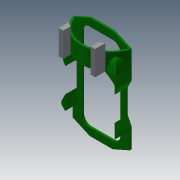
# Autodesk Inventor part: podvozek_dibond
Saved by Autodesk Inventor 2013 (Build 170138000, 138)
## iProperties
Created: 2012-09-03
Part Number: podvozek_dibond
Material: Generic
Document SubType Name: Modeling
Designer: idle-rug
Density: 1 g/cm^3
Author: idle-rug
Autodesk Inventor part; units mm, degrees
ref_plane "YZ Plane" through (0, 0, 0) normal (1, 0, 0) x (0, 1, 0)
ref_plane "XZ Plane" through (0, 0, 0) normal (0, 1, 0) x (-1, 0, 0)
ref_plane "XY Plane" through (0, 0, 0) normal (0, 0, 1) x (1, 0, 0)
sketch "Sketch1" plane through (0, 0, 0) normal (0, 1, 0) x (-1, 0, 0)
  circle A0 centre (24.1, 110.65) radius 0.25
  circle A1 centre (-70.5, 110.65) radius 0.25
  circle A2 centre (-45.6, 89.15) radius 0.25
  circle A3 centre (0, 67.65) radius 0.25
  circle A4 centre (70.5, 42.15) radius 0.25
  circle A5 centre (32.15, 17.15) radius 0.25
  circle A6 centre (60.5, -17.65) radius 0.25
  circle A7 centre (-60.5, -17.65) radius 0.25
  circle A8 centre (24.1, -67.65) radius 0.25
  circle A9 centre (-70.5, -67.65) radius 0.25
  circle A10 centre (-45.6, -89.15) radius 0.25
  circle A11 centre (0, -110.65) radius 0.25
  circle A12 centre (-70.5, -110.65) radius 0.25
  circle A13 centre (70.5, -110.65) radius 0.25
  circle A14 centre (45.6, -89.15) radius 0.25
  circle A15 centre (-24.1, -67.65) radius 0.25
  circle A16 centre (70.5, -67.65) radius 0.25
  circle A17 centre (0, -17.65) radius 0.25
  circle A18 centre (-32.15, 17.15) radius 0.25
  circle A19 centre (-70.5, 42.15) radius 0.25
  circle A20 centre (-70.5, 67.65) radius 0.25
  circle A21 centre (70.5, 67.65) radius 0.25
  circle A22 centre (45.6, 89.15) radius 0.25
  circle A23 centre (-24.1, 110.65) radius 0.25
  circle A24 centre (70.5, 110.65) radius 0.25
  line L0 (75.5, -115.65) -> (75.5, -62.65)
  line L1 (75.5, -62.65) -> (65.5, -42.65)
  line L2 (65.5, -42.65) -> (65.5, 22.15)
  line L3 (65.5, 22.15) -> (75.5, 42.15)
  line L4 (75.5, 42.15) -> (75.5, 115.65)
  line L5 (75.5, 115.65) -> (30.5, 135.65)
  line L6 (30.5, 135.65) -> (-30.5, 135.65)
  line L7 (-30.5, 135.65) -> (-75.5, 115.65)
  line L8 (-75.5, 115.65) -> (-75.5, 42.15)
  line L9 (-75.5, 42.15) -> (-65.5, 22.15)
  line L10 (-65.5, 22.15) -> (-65.5, -42.65)
  line L11 (-65.5, -42.65) -> (-75.5, -62.65)
  line L12 (-75.5, -62.65) -> (-75.5, -115.65)
  line L13 (-75.5, -115.65) -> (-30.5, -135.65)
  line L14 (-30.5, -135.65) -> (30.5, -135.65)
  line L15 (30.5, -135.65) -> (75.5, -115.65)
  circle A25 centre (0, -110.65) radius 2
  circle A26 centre (70.5, -110.65) radius 2
  circle A27 centre (-70.5, -110.65) radius 2
  circle A28 centre (45.6, -89.15) radius 2
  circle A29 centre (-45.6, -89.15) radius 2
  circle A30 centre (70.5, -67.65) radius 2
  circle A31 centre (24.1, -67.65) radius 2
  circle A32 centre (-24.1, -67.65) radius 2
  circle A33 centre (-70.5, -67.65) radius 2
  circle A34 centre (60.5, -17.65) radius 2
  circle A35 centre (0, -17.65) radius 2
  circle A36 centre (-32.15, 17.15) radius 2
  circle A37 centre (-60.5, -17.65) radius 2
  circle A38 centre (32.15, 17.15) radius 2
  circle A39 centre (70.5, 42.15) radius 2
  circle A40 centre (-70.5, 42.15) radius 2
  circle A41 centre (-70.5, 67.65) radius 2
  circle A42 centre (0, 67.65) radius 2
  circle A43 centre (70.5, 67.65) radius 2
  circle A44 centre (45.6, 89.15) radius 2
  circle A45 centre (-45.6, 89.15) radius 2
  circle A46 centre (-70.5, 110.65) radius 2
  circle A47 centre (-24.1, 110.65) radius 2
  circle A48 centre (24.1, 110.65) radius 2
  circle A49 centre (70.5, 110.65) radius 2
  point P0 (0, 0)
  point P1 (0, 0)
  dimension "d0" = 4
  dimension "d1" = 4
  dimension "d2" = 4
  dimension "d3" = 4
  dimension "d4" = 4
  dimension "d5" = 4
  dimension "d6" = 4
  dimension "d7" = 4
  dimension "d8" = 4
  dimension "d9" = 4
  dimension "d10" = 4
  dimension "d11" = 4
  dimension "d12" = 4
  dimension "d13" = 4
  dimension "d14" = 4
  dimension "d15" = 4
  dimension "d16" = 4
  dimension "d17" = 4
  dimension "d18" = 4
  dimension "d19" = 4
  dimension "d20" = 4
  dimension "d21" = 4
  dimension "d22" = 4
  dimension "d23" = 4
  dimension "d24" = 4
  constraints: 50 centre point, 32 end point, 25 coincident
  measures "d0" diameter of A25
  measures "d1" diameter of A26
  measures "d2" diameter of A27
  measures "d3" diameter of A28
  measures "d4" diameter of A29
  measures "d5" diameter of A30
  measures "d6" diameter of A31
  measures "d7" diameter of A32
  measures "d8" diameter of A33
  measures "d9" diameter of A34
  measures "d10" diameter of A35
  measures "d11" diameter of A36
  measures "d12" diameter of A37
  measures "d13" diameter of A38
  measures "d14" diameter of A39
  measures "d15" diameter of A40
  measures "d16" diameter of A41
  measures "d17" diameter of A42
  measures "d18" diameter of A43
  measures "d19" diameter of A44
  measures "d20" diameter of A45
  measures "d21" diameter of A46
  measures "d22" diameter of A47
  measures "d23" diameter of A48
  measures "d24" diameter of A49
extrude "Extrusion1" add sketch "Sketch1" along normal blind 2 contours L15 L14 L13 L12 L11 L10 L9 L8 L7 L6 L5 L4 L3 L2 L1 L0
sketch "Sketch2" plane through (0, 0, 0) normal (0, -1, 0) x (1, 0, 0)
  circle A0 centre (-70.5, 110.65) radius 2 projected
  circle A1 centre (-24.1, 110.65) radius 2 projected
  circle A2 centre (24.1, 110.65) radius 2 projected
  circle A3 centre (70.5, 110.65) radius 2 projected
  circle A4 centre (45.6, 89.15) radius 2 projected
  circle A5 centre (-45.6, 89.15) radius 2 projected
  circle A6 centre (-70.5, 67.65) radius 2 projected
  circle A7 centre (0, 67.65) radius 2 projected
  circle A8 centre (70.5, 67.65) radius 2 projected
  circle A9 centre (70.5, 42.15) radius 2 projected
  circle A10 centre (-70.5, 42.15) radius 2 projected
  circle A11 centre (-32.15, 17.15) radius 2 projected
  circle A12 centre (60.5, -17.65) radius 2 projected
  circle A13 centre (32.15, 17.15) radius 2 projected
  circle A14 centre (0, -17.65) radius 2 projected
  circle A15 centre (-60.5, -17.65) radius 2 projected
  circle A16 centre (70.5, -67.65) radius 2 projected
  circle A17 centre (24.1, -67.65) radius 2 projected
  circle A18 centre (-24.1, -67.65) radius 2 projected
  circle A19 centre (-70.5, -67.65) radius 2 projected
  circle A20 centre (45.6, -89.15) radius 2 projected
  circle A21 centre (-45.6, -89.15) radius 2 projected
  circle A22 centre (70.5, -110.65) radius 2 projected
  circle A23 centre (-70.5, -110.65) radius 2 projected
  circle A24 centre (0, -110.65) radius 2 projected
  line L0 (65.5, 22.15) -> (75.5, 42.15) projected
  line L1 (75.5, 42.15) -> (75.5, 115.65) projected
  line L2 (75.5, 115.65) -> (30.5, 135.65) projected
  line L3 (30.5, 135.65) -> (-30.5, 135.65) projected
  line L4 (-30.5, 135.65) -> (-75.5, 115.65) projected
  line L5 (-75.5, 115.65) -> (-75.5, 42.15) projected
  line L6 (-75.5, 42.15) -> (-65.5, 22.15) projected
  line L7 (-65.5, 22.15) -> (-65.5, -42.65) projected
  line L8 (-65.5, -42.65) -> (-75.5, -62.65) projected
  line L9 (-75.5, -62.65) -> (-75.5, -115.65) projected
  line L10 (-75.5, -115.65) -> (-30.5, -135.65) projected
  line L11 (-30.5, -135.65) -> (30.5, -135.65) projected
  line L12 (30.5, -135.65) -> (75.5, -115.65) projected
  line L13 (75.5, -115.65) -> (75.5, -62.65) projected
  line L14 (75.5, -62.65) -> (65.5, -42.65) projected
  line L15 (65.5, -42.65) -> (65.5, 22.15) projected
  point P0 (0, 0)
extrude "Extrusion2" add sketch "Sketch2" along normal blind 1.3
sketch "Sketch3" plane through (0, -1.3, 0) normal (0, -1, 0) x (1, 0, 0)
  circle A0 centre (0, -110.65) radius 2 projected
  circle A1 centre (-45.6, -89.15) radius 2 projected
  circle A2 centre (45.6, -89.15) radius 2 projected
  circle A3 centre (-24.1, -67.65) radius 2 projected
  circle A4 centre (24.1, -67.65) radius 2 projected
  circle A5 centre (0, 67.65) radius 2 projected
  circle A6 centre (-45.6, 89.15) radius 2 projected
  circle A7 centre (45.6, 89.15) radius 2 projected
  circle A8 centre (24.1, 110.65) radius 2 projected
  circle A9 centre (-24.1, 110.65) radius 2 projected
  line L0 (-75.5, 115.65) -> (-75.5, 42.15) projected
  line L1 (75.5, 115.65) -> (-75.5, 115.65)
  line L2 (-75.5, 115.65) -> (-75.5, 105.65)
  line L3 (-75.5, 105.65) -> (75.5, 105.65)
  line L4 (75.5, 105.65) -> (75.5, 115.65)
  line L5 (75.5, 72.65) -> (-75.5, 72.65)
  line L6 (-75.5, 72.65) -> (-75.5, 62.65)
  line L7 (-75.5, 62.65) -> (75.5, 62.65)
  line L8 (75.5, 62.65) -> (75.5, 72.65)
  line L9 (75.5, 72.65) -> (-75.5, 62.65) construction
  line L10 (-75.5, 72.65) -> (75.5, 62.65) construction
  line L11 (50.6, 115.65) -> (40.6, 115.65)
  line L12 (40.6, 115.65) -> (40.6, 62.65)
  line L13 (40.6, 62.65) -> (50.6, 62.65)
  line L14 (50.6, 62.65) -> (50.6, 115.65)
  line L15 (50.6, 115.65) -> (40.6, 62.65) construction
  line L16 (40.6, 115.65) -> (50.6, 62.65) construction
  line L17 (-40.6, 115.65) -> (-50.6, 115.65)
  line L18 (-50.6, 115.65) -> (-50.6, 62.65)
  line L19 (-50.6, 62.65) -> (-40.6, 62.65)
  line L20 (-40.6, 62.65) -> (-40.6, 115.65)
  line L21 (-40.6, 115.65) -> (-50.6, 62.65) construction
  line L22 (-50.6, 115.65) -> (-40.6, 62.65) construction
  line L23 (-75.5, -72.65) -> (75.5, -72.65)
  line L24 (75.5, -72.65) -> (75.5, -62.65)
  line L25 (75.5, -62.65) -> (-75.5, -62.65)
  line L26 (-75.5, -62.65) -> (-75.5, -72.65)
  line L27 (-75.5, -72.65) -> (75.5, -62.65) construction
  line L28 (75.5, -72.65) -> (-75.5, -62.65) construction
  line L29 (75.5, -105.65) -> (-75.5, -105.65)
  line L30 (-75.5, -105.65) -> (-75.5, -115.65)
  line L31 (-75.5, -115.65) -> (75.5, -115.65)
  line L32 (75.5, -115.65) -> (75.5, -105.65)
  line L33 (75.5, -105.65) -> (-75.5, -115.65) construction
  line L34 (-75.5, -105.65) -> (75.5, -115.65) construction
  line L35 (50.6, -62.65) -> (40.6, -62.65)
  line L36 (40.6, -62.65) -> (40.6, -115.65)
  line L37 (40.6, -115.65) -> (50.6, -115.65)
  line L38 (50.6, -115.65) -> (50.6, -62.65)
  line L39 (50.6, -62.65) -> (40.6, -115.65) construction
  line L40 (40.6, -62.65) -> (50.6, -115.65) construction
  line L41 (-40.6, -62.65) -> (-50.6, -62.65)
  line L42 (-50.6, -62.65) -> (-50.6, -115.65)
  line L43 (-50.6, -115.65) -> (-40.6, -115.65)
  line L44 (-40.6, -115.65) -> (-40.6, -62.65)
  line L45 (-40.6, -62.65) -> (-50.6, -115.65) construction
  line L46 (-50.6, -62.65) -> (-40.6, -115.65) construction
  line L47 (30.5, 135.65) -> (75.5, 115.65) projected
  line L48 (-50.6, 115.65) -> (50.6, 115.65)
  line L49 (50.6, 115.65) -> (50.6, -115.65)
  line L50 (50.6, -115.65) -> (-50.6, -115.65)
  line L51 (-50.6, -115.65) -> (-50.6, 115.65)
  point P0 (0, 0)
  point P1 (0, -67.65)
  dimension "d29" = 10
  dimension "d30" = 10
  dimension "d31" = 10
  dimension "d32" = 10
  dimension "d33" = 10
  dimension "d34" = 10
  constraints: 100 end point, 18 parallel, 14 midpoint, 9 horizontal, 9 perpendicular, 6 point on line
  measures "d29" distance of L2.end L1.end
  measures "d30" distance of L6.end L5.end
  measures "d31" distance of L13.end L12.end
  measures "d32" distance of L19.end L18.end
  measures "d33" distance of L37.end L36.end
  measures "d34" distance of L43.end L42.end
extrude "Extrusion3" cut sketch "Sketch3" against normal blind 3.3 contours A0 | A1 | A2 | A3 | A4 | A5 | A6 | A7 | A8 | A9 | L1 L20 L3 L18 | L3 L20 L5 L18 | L1 L12 L3 L20 | L5 L20 L7 L18 | L3 L12 L5 L20 | L1 L14 L3 L12 | L7 L49 L25 L51 | L5 L12 L7 L20 | L3 L14 L5 L12 | L25 L44 L23 L42 | L5 L14 L7 L12 | L25 L36 L23 L44 | L23 L44 L29 L42 | L25 L38 L23 L36 | L23 L36 L29 L44 | L29 L44 L31 L42 | L23 L38 L29 L36 | L29 L36 L31 L44 | L29 L38 L31 L36
fillet "Fillet1" radius 20 4 edges at (-50.6, 0.35, 115.65) (-50.6, 0.35, -115.65) (50.6, 0.35, -115.65) (50.6, 0.35, 115.65)
sketch "Sketch5" plane through (0, -1.3, 0) normal (0, -1, 0) x (1, 0, 0)
  circle A0 centre (-70.5, -110.65) radius 2 projected
  circle A1 centre (70.5, -110.65) radius 2 projected
  circle A2 centre (-70.5, -67.65) radius 2 projected
  circle A3 centre (70.5, -67.65) radius 2 projected
  circle A4 centre (-70.5, 42.15) radius 2 projected
  circle A5 centre (70.5, 42.15) radius 2 projected
  circle A6 centre (70.5, 67.65) radius 2 projected
  circle A7 centre (-70.5, 67.65) radius 2 projected
  circle A8 centre (70.5, 110.65) radius 2 projected
  circle A9 centre (-70.5, 110.65) radius 2 projected
  point P0 (0, 0)
extrude "Extrusion4" add sketch "Sketch5" against normal blind 3
sketch "Sketch6" plane through (0, 2, 0) normal (0, 1, 0) x (1, 0, 0)
  circle A0 centre (60.5, 17.65) radius 2 projected
  circle A1 centre (-60.5, 17.65) radius 2 projected
  point P0 (0, 0)
extrude "Extrusion5" add sketch "Sketch6" against normal blind 3.3
sketch "Sketch7" plane through (0, -1.3, 0) normal (0, -1, 0) x (1, 0, 0)
  line L0 (-30.6, 115.65) -> (30.6, 115.65) projected
  arc A0 (50.6, 95.65) -> (30.6, 115.65) centre (30.6, 95.65) ccw projected
  line L1 (50.6, 95.65) -> (50.6, -95.65) projected
  arc A1 (30.6, -115.65) -> (50.6, -95.65) centre (30.6, -95.65) ccw projected
  line L2 (30.6, -115.65) -> (-30.6, -115.65) projected
  arc A2 (-50.6, -95.65) -> (-30.6, -115.65) centre (-30.6, -95.65) ccw projected
  line L3 (-50.6, -95.65) -> (-50.6, 95.65) projected
  arc A3 (-30.6, 115.65) -> (-50.6, 95.65) centre (-30.6, 95.65) ccw projected
  line L4 (65.5, 22.15) -> (75.5, 42.15) projected
  line L5 (75.5, 42.15) -> (75.5, 115.65) projected
  line L6 (75.5, 115.65) -> (30.5, 135.65) projected
  line L7 (30.5, 135.65) -> (-30.5, 135.65) projected
  line L8 (-30.5, 135.65) -> (-75.5, 115.65) projected
  line L9 (-75.5, 115.65) -> (-75.5, 42.15) projected
  line L10 (-75.5, 42.15) -> (-65.5, 22.15) projected
  line L11 (-65.5, 22.15) -> (-65.5, -42.65) projected
  line L12 (-65.5, -42.65) -> (-75.5, -62.65) projected
  line L13 (-75.5, -62.65) -> (-75.5, -115.65) projected
  line L14 (-75.5, -115.65) -> (-30.5, -135.65) projected
  line L15 (-30.5, -135.65) -> (30.5, -135.65) projected
  line L16 (30.5, -135.65) -> (75.5, -115.65) projected
  line L17 (75.5, -115.65) -> (75.5, -62.65) projected
  line L18 (75.5, -62.65) -> (65.5, -42.65) projected
  line L19 (65.5, -42.65) -> (65.5, 22.15) projected
  point P0 (0, 0)
extrude "Extrusion6" add sketch "Sketch7" along normal blind 1.7
sketch "Sketch9" plane through (-30.5, 2, 135.65) normal (0, 0, 1) x (1, 0, 0)
  line L0 (106, 0) -> (101, 0)
  line L1 (-45, -5) -> (-40, -5)
  line L2 (106, -5) -> (101, -5)
  arc A0 (-45, -5) -> (106, -5) centre (30.5, 21.4528) ccw
  arc A1 (-40, -5) -> (101, -5) centre (30.5, 21.4528) ccw
  line L3 (106, -5) -> (101, -5)
  line L4 (-45, -5) -> (-40, -5)
  line L5 (-45, -5) -> (-35, -5) projected
  arc A2 (-40, -5) -> (101, -5) centre (30.5, 21.4528) ccw
  point P0 (-45, 0)
  dimension "d46" = 80
  constraints: 10 end point, 7 point on circle, 3 centre point, 3 concentric, 2 collinear, 1 midpoint
  measures "d46" radius of A0
extrude "Extrusion7" add sketch "Sketch9" against normal blind 65
sketch "Sketch10" plane through (-30.5, 2, 135.65) normal (0, 0, 1) x (1, 0, 0)
  arc A0 (-45, -5) -> (106, -5) centre (30.5, 21.4528) ccw projected
  line L0 (106, -5) -> (101, -5) projected
  arc A1 (-40, -5) -> (101, -5) centre (30.5, 21.4528) ccw projected
  line L1 (-40, -5) -> (-45, -5) projected
  point P0 (30.5, -2)
extrude "Extrusion8" cut sketch "Sketch10" against normal blind 20
sketch "Sketch11" plane through (0, -3, 0) normal (0, -1, 0) x (1, 0, 0)
  line L0 (75.5, -115.65) -> (75.5, -62.65) projected
  line L1 (75.5, -62.65) -> (65.5, -42.65) projected
  line L2 (-30.6, 115.65) -> (30.6, 115.65) projected
  line L3 (65.5, -42.65) -> (65.5, -95.65)
  line L4 (65.5, -95.65) -> (75.5, -95.65)
  line L5 (75.5, -62.65) -> (75.5, -95.65)
  line L6 (65.5, -42.65) -> (75.5, -62.65)
  line L7 (65.5, -42.65) -> (75.5, -62.65)
  line L8 (0, 0) -> (0, -83)
  line L9 (-65.5, -42.65) -> (-65.5, -95.65)
  line L10 (-65.5, -95.65) -> (-75.5, -95.65)
  line L11 (-75.5, -62.65) -> (-75.5, -95.65)
  line L12 (-65.5, -42.65) -> (-75.5, -62.65)
  dimension "d51" = 53
  constraints: 20 end point, 3 collinear, 2 perpendicular, 2 symmetric about line, 1 parallel, 1 point on line
  measures "d51" distance of L1.end L3.end
extrude "Extrusion9" add sketch "Sketch11" along normal blind 30
sketch "Sketch12" plane through (0, -3, 0) normal (0, -1, 0) x (1, 0, 0)
  line L0 (65.5, -95.65) -> (65.5, -42.65) projected
  line L1 (65.5, -42.65) -> (65.5, 22.15) projected
  line L2 (65.5, 22.15) -> (75.5, 42.15) projected
  line L3 (75.5, 42.15) -> (75.5, 70.65) projected
  line L4 (75.5, 70.65) -> (70.5, 70.65) projected
  line L5 (-75.5, 70.65) -> (-75.5, 42.15) projected
  line L6 (-75.5, 42.15) -> (-65.5, 22.15) projected
  line L7 (-65.5, 22.15) -> (-65.5, -42.65) projected
  line L8 (-65.5, -42.65) -> (-65.5, -95.65) projected
  line L9 (-65.5, -95.65) -> (-75.5, -95.65) projected
  line L10 (-75.5, -95.65) -> (-75.5, -115.65) projected
  line L11 (-75.5, -115.65) -> (-30.5, -135.65) projected
  line L12 (-30.5, -135.65) -> (30.5, -135.65) projected
  line L13 (30.5, -135.65) -> (75.5, -115.65) projected
  line L14 (75.5, -115.65) -> (75.5, -95.65) projected
  line L15 (75.5, -95.65) -> (65.5, -95.65) projected
  line L16 (-30.6, 115.65) -> (30.6, 115.65) projected
  line L17 (65.5, 23) -> (65.5, 70.65)
  line L18 (75.5, 70.65) -> (65.5, 70.65)
  line L19 (-75.5, 70.65) -> (75.5, 70.65) projected
  line L20 (75.5, 70.65) -> (75.5, 42.15)
  line L21 (75.5, 42.15) -> (65.5, 22.15)
  line L22 (65.5, 22) -> (65.5, 23)
  line L23 (-65.5, 22.15) -> (-75.5, 42.15)
  line L24 (-75.5, 42.15) -> (-75.5, 70.65)
  line L25 (-75.5, 70.65) -> (-65.5, 70.65)
  line L26 (-65.5, 70.65) -> (-65.5, 22.15)
  point P0 (-70.5, 70.65)
  point P1 (0, 0)
  constraints: 19 end point, 4 point on line, 3 collinear, 2 perpendicular, 1 parallel
extrude "Extrusion10" add sketch "Sketch12" along normal blind 30 contours L22 L17 L18 L4 L3 L2 | L26 L6 L5 L19
sketch "Sketch13" plane through (65.5, -33, 70.65) normal (0, 0, 1) x (1, 0, 0)
  arc A0 (0, 10.5208) -> (10, 30) centre (-65.5, 56.4528) ccw projected
  line L0 (0, 10.5208) -> (0, 0) projected
  line L1 (10, 0) -> (0, 0) projected
  line L2 (10, 30) -> (10, 0) projected
  point P0 (-65.5, 33)
extrude "Extrusion11" add sketch "Sketch13" along normal blind 35
sketch "Sketch14" plane through (0, -33, 0) normal (0, -1, 0) x (1, 0, 0)
  line L0 (-5, 75.5) -> (5, 75.5)
  line L1 (-75.5, 70.65) -> (-75.5, 62.65)
  line L2 (75.5, 62.65) -> (75.5, 70.65)
  line L3 (75.5, 42.15) -> (75.5, 105.65) projected
  arc A0 (-41.3014, 70.65) -> (-75.5, 45.15) centre (0, -20.4225) ccw
  arc A1 (75.5, 45.15) -> (41.3014, 70.65) centre (0, -20.4225) ccw
  line L4 (-75.5, 70.65) -> (-41.3014, 70.65)
  line L5 (41.3014, 70.65) -> (75.5, 70.65)
  line L6 (75.5, 70.65) -> (75.5, 45.15)
  line L7 (-75.5, 70.65) -> (-75.5, 45.15)
  point P0 (0, 0)
  point P1 (-75.5, 42.15)
  dimension "d58" = 3
  dimension "d59" = 3
  constraints: 14 end point, 5 point on circle, 2 centre point, 1 collinear, 1 perpendicular, 1 point on line
  measures "d58" distance of L3.start L6.end
  measures "d59" distance of point (-75.5, 42.15) L7.end
extrude "Extrusion12" add sketch "Sketch14" along normal blind 6.2
sketch "Sketch15" plane through (56.6841, -33, 70.65) normal (0, 0, 1) x (1, 0, 0)
  arc A0 (-6.9384, -6.2) -> (0, 0) centre (-56.6841, 56.4528) ccw projected
  line L0 (18.8159, -6.2) -> (-6.9384, -6.2) projected
  line L1 (18.8159, 0) -> (18.8159, -6.2) projected
  line L2 (8.8159, 0) -> (18.8159, 0) projected
  line L3 (8.8159, 0) -> (0, 0) projected
  line L4 (8.8159, 10.5208) -> (8.8159, 0)
  line L5 (8.8159, 30) -> (8.8159, 0) projected
  line L6 (0, 0) -> (8.8159, 0)
  arc A1 (0, 0) -> (8.8159, 10.5208) centre (-51.062, 51.7418) ccw
  point P0 (-56.6841, 33)
  constraints: 4 end point, 3 point on circle, 2 collinear, 1 centre point
extrude "Extrusion13" add sketch "Sketch15" along normal blind 35
sketch "Sketch16" plane through (0, -39.2, 0) normal (0, -1, 0) x (1, 0, 0)
  line L0 (-41.3014, 70.65) -> (-41.7687, 70.65) projected
  line L1 (-49.7456, 70.65) -> (-41.7687, 70.65) projected
  line L2 (-49.7456, 70.65) -> (-75.5, 70.65) projected
  line L3 (-75.5, 70.65) -> (-75.5, 45.15) projected
  arc A0 (-41.3014, 70.65) -> (-75.5, 45.15) centre (0, -20.4225) ccw projected
  point P0 (0, 0)
extrude "Extrusion14" cut sketch "Sketch16" against normal blind 6.2
sketch "Sketch17" plane through (0, -33, 0) normal (0, -1, 0) x (1, 0, 0)
  line L0 (-75.5, 70.65) -> (-75.5, 42.15) projected
  line L1 (-75.5, 42.15) -> (-65.5, 22.15) projected
  line L2 (-65.5, 22.15) -> (-65.5, 70.65) projected
  line L3 (-75.5, 70.65) -> (-65.5, 70.65) projected
  point P0 (0, 0)
extrude "Extrusion15" cut sketch "Sketch17" against normal blind 30
sketch "Sketch18" plane through (0, -3, 0) normal (0, -1, 0) x (1, 0, 0)
  line L0 (-70.5, 115.65) -> (-70.5, 70.65) projected
  line L1 (-75.5, 42.15) -> (-75.5, 70.65) projected
  line L2 (-65.5, 22.15) -> (-75.5, 42.15) projected
  line L3 (-65.5, 22.15) -> (-65.5, 105.65)
  line L4 (-65.5, 105.65) -> (-75.5, 105.65)
  line L5 (-75.5, 115.65) -> (-75.5, 70.65) projected
  line L6 (41.7687, 70.65) -> (-70.5, 70.65) projected
  line L7 (-65.5, 70.65) -> (-75.5, 70.65)
  point P0 (0, 0)
  dimension "d88" = 83.5
  constraints: 6 end point, 3 point on line, 2 perpendicular, 1 parallel
  measures "d88" distance of L2.start L3.end
extrude "Extrusion16" add sketch "Sketch18" along normal blind 30 contours L6 L3 L2 L1 L7
sketch "Sketch19" plane through (-75.5, -33, 70.65) normal (0, 0, 1) x (1, 0, 0)
  arc A0 (0, 30) -> (10, 10.5208) centre (75.5, 56.4528) ccw projected
  line L0 (0, 30) -> (0, 0) projected
  line L1 (10, 0) -> (0, 0) projected
  line L2 (10, 10.5208) -> (10, 0) projected
  arc A1 (0, 30) -> (151, 30) centre (75.5, 56.4528) ccw projected
  arc A2 (10, 10.5208) -> (18.8159, 0) centre (75.5, 56.4528) ccw
  line L3 (10, 10.5208) -> (10, 0)
  line L4 (18.8159, 0) -> (10, 0)
  point P0 (75.5, 33)
  constraints: 4 end point, 3 point on circle, 1 centre point, 1 collinear, 1 concentric
extrude "Extrusion17" add sketch "Sketch19" along normal blind 35
sketch "Sketch20" plane through (0, -33, 0) normal (0, -1, 0) x (1, 0, 0)
  line L0 (-75.5, 42.15) -> (-75.5, 105.65) projected
  line L1 (-75.5, 42.15) -> (-75.5, 45.15)
  line L2 (-75.5, 42.15) -> (-75.5, 115.65) projected
  line L3 (75.5, 42.15) -> (75.5, 45.15)
  line L4 (75.5, 115.65) -> (75.5, 42.15) projected
  line L5 (41.7687, 70.65) -> (-65.5, 70.65) projected
  line L6 (-41.5716, 70.65) -> (-75.5, 70.65)
  line L7 (-75.5, 70.65) -> (-75.5, 45.15)
  arc A0 (-41.5716, 70.65) -> (-75.5, 45.15) centre (0, -19.9834) ccw
  point P0 (0, 0)
  dimension "d93" = 3
  dimension "d94" = 3
  constraints: 8 end point, 4 point on line, 2 perpendicular, 2 point on circle, 1 centre point
  measures "d93" distance of L0.start L1.end
  measures "d94" distance of L3.start L3.end
extrude "Extrusion18" add sketch "Sketch20" along normal blind 5
sketch "Sketch21" plane through (-75.5, -33, 70.65) normal (0, 0, 1) x (1, 0, 0)
  arc A0 (18.8159, 0) -> (24.2794, -5) centre (75.5, 56.4528) ccw projected
  line L0 (10, 0) -> (18.8159, 0) projected
  line L1 (0, 0) -> (10, 0) projected
  line L2 (0, 0) -> (0, -5) projected
  line L3 (24.2794, -5) -> (0, -5) projected
  point P0 (75.5, 33)
extrude "Extrusion19" add sketch "Sketch21" along normal blind 35
sketch "Sketch22" plane through (0, -38, 0) normal (0, -1, 0) x (1, 0, 0)
  line L0 (-75.5, 45.15) -> (-75.5, 105.65) projected
  arc A0 (-41.5716, 70.65) -> (-75.5, 45.15) centre (0, -19.9834) ccw projected
  line L1 (-41.5716, 70.65) -> (-43.515, 70.65) projected
  line L2 (-51.2206, 70.65) -> (-43.515, 70.65) projected
  line L3 (-51.2206, 105.65) -> (-51.2206, 70.65) projected
  line L4 (-75.5, 105.65) -> (-51.2206, 105.65) projected
  point P0 (0, 0)
extrude "Extrusion20" add sketch "Sketch22" along normal blind 1.2
chamfer "Chamfer8" distance 12.85 angle 45 4 edges at (62.6228, -39.2, 105.65) (75.5, -21.1, 105.65) (-63.3603, -39.2, 105.65) (-75.5, -21.1, 105.65)
chamfer "Chamfer9" distance 10 angle 45 4 edges at (-63.3603, -39.2, 92.8) (-75.5, -21.1, 92.8) (62.6228, -39.2, 92.8) (75.5, -21.1, 92.8)
chamfer "Chamfer10" distance 10 angle 45 4 edges at (62.6228, -39.2, 82.8) (75.5, -21.1, 82.8) (-75.5, -21.1, 82.8) (-63.3603, -39.2, 82.8)
fillet "Fillet6" radius 21 12 edges at (62.6228, -39.2, 72.8) (75.5, -21.1, 72.8) (62.9452, -35.3732, 92.0388) (71.6732, -23.7292, 92.0388) (62.9904, -32.1289, 99.8711) (68.4289, -25.0593, 99.8711) (-63.3603, -39.2, 72.8) (-75.5, -21.1, 72.8) (-62.9452, -35.3732, 92.0388) (-71.6732, -23.7292, 92.0388) (-62.9837, -32.1289, 99.8711) (-68.4289, -25.0593, 99.8711)
sketch "Sketch23" plane through (0, -33, 0) normal (0, -1, 0) x (1, 0, 0)
  line L0 (65.5, -42.65) -> (65.5, -95.65) projected
  line L1 (65.5, -95.65) -> (75.5, -95.65) projected
  line L2 (75.5, -62.65) -> (75.5, -70.65)
  line L3 (-75.5, -62.65) -> (-75.5, -95.65) projected
  line L4 (65.5, -80.6404) -> (65.5, -95.65)
  line L5 (65.5, -95.65) -> (75.5, -95.65)
  line L6 (75.5, -95.65) -> (75.5, -70.65)
  line L7 (-75.5, -70.65) -> (-75.5, -95.65)
  line L8 (-75.5, -95.65) -> (-65.5, -95.65) projected
  line L9 (-65.5, -95.65) -> (-75.5, -95.65)
  line L10 (-65.5, -95.65) -> (-65.5, -80.6404)
  line L11 (-65.5, -95.65) -> (-65.5, -42.65) projected
  arc A0 (-75.5, -70.65) -> (-65.5, -80.6404) centre (0, -5.0775) ccw
  arc A1 (65.5, -80.6404) -> (75.5, -70.65) centre (0, -5.0775) ccw
  point P0 (0, 0)
  dimension "d117" = 8
  constraints: 14 end point, 4 point on circle, 3 perpendicular, 3 point on line, 2 centre point, 1 parallel
  measures "d117" distance of L2.start L2.end
extrude "Extrusion21" cut sketch "Sketch23" against normal blind 30
sketch "Sketch24" plane through (-30.5, 2, 115.65) normal (0, 0, 1) x (1, 0, 0)
  arc A0 (-45, -5) -> (106, -5) centre (30.5, 21.4528) ccw projected
  line L0 (-10.8, -69.51) -> (-5.8, -69.51)
  line L1 (-10.8, -69.51) -> (-5.8, -69.51)
  line L2 (71.8, -69.51) -> (66.8, -69.51)
  line L3 (-10.8, -69.51) -> (-17.8, -69.51)
  line L4 (78.8, -41.51) -> (78.8, -69.51)
  line L5 (78.8, -69.51) -> (71.8, -69.51)
  arc A1 (-17.8, -42.3211) -> (-5.8, -49.8375) centre (30.5, 21.4528) ccw
  arc A2 (-19.2456, -41.2) -> (80.2456, -41.2) centre (30.5, 21.4528) ccw projected
  arc A3 (66.8, -49.8375) -> (78.8, -42.3211) centre (28.427, 24.7623) ccw
  line L6 (78.8, -42.3211) -> (78.8, -69.51)
  line L7 (78.8, -69.51) -> (66.8, -69.51)
  line L8 (66.8, -69.51) -> (66.8, -49.8375)
  line L9 (-5.8, -49.8375) -> (-5.8, -69.51)
  line L10 (-5.8, -69.51) -> (-17.8, -69.51)
  line L11 (-17.8, -69.51) -> (-17.8, -42.3211)
  point P0 (30.5, -2)
  point P1 (30.5, -55.51)
  dimension "d121" = 82.6
  dimension "d123" = 5
  dimension "d130" = 7
  dimension "d131" = 28
  constraints: 24 end point, 8 point on circle, 3 horizontal, 2 centre point, 2 perpendicular, 1 point on line
  measures "d121" distance of L2.start L0.start
  measures "d123" distance of L0.start L0.end
  measures "d130" distance of L4.end L5.end
  measures "d131" distance of L4.start L4.end
extrude "Extrusion22" add sketch "Sketch24" against normal blind 45 contours A0 L9 L0 L3 L11 | A0 L4 L5 L2 L8
sketch "Sketch25" plane through (-30.5, 2, 115.65) normal (0, 0, 1) x (1, 0, 0)
  line L0 (-17.8, -42.3211) -> (-17.8, -69.51) projected
  line L1 (66.8, -49.8375) -> (66.8, -69.51) projected
  line L2 (66.8, -69.51) -> (78.8, -69.51) projected
  arc A0 (-17.8, -42.3211) -> (-5.8, -49.8375) centre (30.5, 21.4528) ccw
  arc A1 (66.8, -49.8375) -> (78.8, -42.3211) centre (30.5, 21.4528) ccw
  line L3 (-17.8, -42.3211) -> (-17.8, -69.51)
  line L4 (-17.8, -69.51) -> (-17.8, -42.3211) projected
  line L5 (-5.8, -69.51) -> (-17.8, -69.51)
  line L6 (-5.8, -49.8375) -> (-5.8, -69.51)
  line L7 (-5.8, -49.8375) -> (-5.8, -69.51) projected
  line L8 (66.8, -49.8375) -> (66.8, -69.51)
  line L9 (78.8, -69.51) -> (66.8, -69.51)
  line L10 (78.8, -69.51) -> (66.8, -69.51) projected
  line L11 (78.8, -42.3211) -> (78.8, -69.51)
  point P0 (30.5, -2)
  constraints: 12 end point, 5 point on circle, 4 collinear, 2 centre point, 2 perpendicular, 1 point on line
extrude "Extrusion23" add sketch "Sketch25" along normal blind 20
body "Solid1"
